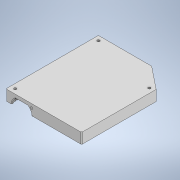
# Autodesk Inventor part: BoxDeckel
Saved by Autodesk Inventor 2020 (Build 240168000, 168)
## iProperties
Created: 2020-04-10
Part Number: BoxDeckel
Material: Generisch
Document SubType Name: Modeling
Designer: Windooof
Density: 1 g/cm^3
Appearance: Vorgabe
Author: Windooof
Autodesk Inventor part; units mm, degrees
ref_plane "YZ Plane" through (0, 0, 0) normal (1, 0, 0) x (0, 1, 0)
ref_plane "XZ Plane" through (0, 0, 0) normal (0, 1, 0) x (-1, 0, 0)
ref_plane "XY Plane" through (0, 0, 0) normal (0, 0, 1) x (1, 0, 0)
sketch "SketchBase" plane through (0, 0, 0) normal (0, 1, 0) x (-1, 0, 0)
  line L0 (45, 55) -> (-45, 55)
  line L1 (-45, 55) -> (-45, -33.701562)
  line L2 (-18.376953, -55) -> (45, -55)
  line L3 (45, -55) -> (45, 55)
  line L4 (63, 0) -> (-63, 0) construction
  line L5 (0, -77) -> (0, 77) construction
  line L6 (42.5, 52.5) -> (-42.5, 52.5)
  line L7 (-42.5, 52.5) -> (-42.5, -32.5)
  line L8 (-17.5, -52.5) -> (42.5, -52.5)
  line L9 (42.5, -52.5) -> (42.5, 52.5)
  line L10 (0.5, 12.5) -> (7.5, 12.5)
  line L11 (0.5, 5.5) -> (0.5, 12.5)
  line L12 (7.5, 5.5) -> (0.5, 5.5)
  line L13 (0.5, 5.5) -> (7.5, 5.5)
  line L14 (0.5, 3.5) -> (0.5, 5.5)
  line L15 (9.5, 12.5) -> (9.5, 3.5)
  line L16 (9.5, 3.5) -> (0.5, 3.5)
  line L17 (7.5, 12.5) -> (9.5, 12.5)
  line L18 (7.5, 12.5) -> (7.5, 5.5)
  line L19 (7.5, 5.5) -> (7.5, 12.5)
  line L20 (2.5, 44.5) -> (7.5, 44.5)
  line L21 (7.5, 44.5) -> (9.5, 44.5)
  line L22 (7.5, 49.5) -> (7.5, 5.5)
  line L23 (2.5, 49.5) -> (2.5, 44.5)
  line L24 (9.5, 44.5) -> (9.5, 49.5)
  line L25 (7.5, 44.5) -> (7.5, 49.5)
  line L26 (7.5, 49.5) -> (7.5, 44.5)
  line L27 (7.5, 49.5) -> (2.5, 49.5)
  line L28 (-42.5, 49.5) -> (7.5, 49.5)
  line L29 (7.5, 5.5) -> (-42.5, 5.5)
  line L30 (-42.5, 5.5) -> (-42.5, 49.5)
  line L31 (-42.5, 49.5) -> (-36.5, 49.5)
  line L32 (-36.5, 49.5) -> (-36.5, 43.5)
  line L33 (-36.5, 43.5) -> (-42.5, 43.5)
  line L34 (-42.5, 43.5) -> (-42.5, 49.5)
  line L35 (-37.5, 5.5) -> (-37.5, 10.5)
  line L36 (-37.5, 5.5) -> (-37.5, 3.5)
  line L37 (-37.5, 10.5) -> (-42.5, 10.5)
  line L38 (-42.5, 10.5) -> (-42.5, 5.5)
  line L39 (-42.5, 5.5) -> (-37.5, 5.5)
  line L40 (-42.5, 5.5) -> (-37.5, 5.5)
  line L41 (-37.5, 3.5) -> (-42.5, 3.5)
  line L42 (-42.5, 3.5) -> (-42.5, 5.5)
  line L43 (-36.5, 49.5) -> (-42.5, 49.5)
  line L44 (-42.5, 49.5) -> (-42.5, 52.5)
  line L45 (-42.5, 52.5) -> (-36.5, 52.5)
  line L46 (-36.5, 52.5) -> (-36.5, 49.5)
  line L47 (2.5, 49.5) -> (2.5, 52.5)
  line L48 (2.5, 52.5) -> (9.5, 52.5)
  line L49 (9.5, 52.5) -> (9.5, 49.5)
  line L50 (-17.5, -52.5) -> (-42.5, -32.5)
  line L51 (-45, -33.701562) -> (-18.376953, -55)
  line L52 (0, -107.8) -> (0, 107.8)
  line L53 (88.2, 0) -> (-88.2, 0)
  point P0 (0, 0)
  point P1 (0, 0)
  point P2 (-45, -55)
  point P3 (-42.5, -52.5)
  dimension "d0" = 110
  dimension "d1" = 90
  dimension "d2" = 2.5
  dimension "d3" = 2.5
  dimension "d4" = 44
  dimension "d5" = 50
  dimension "d6" = 6
  dimension "d7" = 6
  dimension "d8" = 7
  dimension "d9" = 7
  dimension "d10" = 5
  dimension "d11" = 5
  dimension "d12" = 5
  dimension "d13" = 5
  dimension "d14" = 2
  dimension "d15" = 2
  dimension "d16" = 0
  dimension "d17" = 3
  dimension "d18" = 25
  dimension "d19" = 20
  dimension "d20" = 2.5
  constraints: 104 end point, 20 parallel, 13 perpendicular, 11 horizontal, 8 collinear, 5 point on line, 4 other
  measures "d0" distance of L3.start L0.start
  measures "d1" distance of L0.start L0.end
  measures "d2" distance between parallel lines of L0 L6
  measures "d3" distance between parallel lines of L3 L9
  measures "d4" distance of L27.start L12.start
  measures "d5" distance of L12.start L30.start
  measures "d6" distance of L32.start L32.end
  measures "d7" distance of L32.end L33.end
  measures "d8" distance of L10.start L10.end
  measures "d9" distance of L11.start L10.start
  measures "d10" distance of L23.end L21.start
  measures "d11" distance of L27.end L23.end
  measures "d12" distance of L35.start L35.end
  measures "d13" distance of L35.end L38.start
  measures "d14" distance between parallel lines of L16 L13
  measures "d15" distance between parallel lines of L22 L15
  measures "d16" distance between parallel lines of L7 L30
  measures "d17" distance between parallel lines of L6 L28
  measures "d18" distance of L8.start point (-42.5, -52.5)
  measures "d19" distance of L7.end point (-42.5, -52.5)
  measures "d20" distance between parallel lines of L50 L51
extrude "Base" add sketch "SketchBase" along normal blind 2.5
extrude "Walls" add sketch "SketchBase" against normal blind 10 contours L3 L53 L9 L6 L52 L0 | L52 L6 L7 L53 L1 L0 | L3 L2 L52 L8 L9 L53 | L53 L7 L50 L8 L52 L2 L51 L1
sketch "SketchMounts" plane through (0, 0, 0) normal (0, -1, 0) x (1, 0, 0)
  line L0 (-36.5, -46.5) -> (-36.5, -52.5)
  circle A0 centre (-39.5, -49.5) radius 1.5
  line L1 (-42.5, -46.5) -> (-36.5, -46.5)
  line L2 (-36.5, -52.5) -> (-42.5, -46.5) construction
  line L3 (-36.5, -52.5) -> (-42.5, -52.5)
  line L4 (-36.5, -46.5) -> (-42.5, -52.5) construction
  line L5 (-42.5, -52.5) -> (-42.5, -46.5)
  line L6 (36.232693, -29.487776) -> (42.5, -25.843142)
  circle A1 centre (39.5, -31.058125) radius 1.5
  line L7 (42.5, -32.5) -> (36.232693, -29.487776) construction
  line L8 (37.301867, -36.658506) -> (36.232693, -29.487776)
  line L9 (42.5, -32.5) -> (37.301867, -36.658506)
  line L10 (42.5, -25.843142) -> (42.5, -32.5)
  line L11 (-36.5, 52.5) -> (-42.5, 52.5)
  line L12 (-36.5, 46.5) -> (-36.5, 52.5)
  circle A2 centre (-39.5, 49.5) radius 1.5
  line L13 (-42.5, 46.5) -> (-36.5, 46.5)
  line L14 (-42.5, 52.5) -> (-42.5, 46.5)
  line L15 (-42.5, 52.5) -> (-36.5, 46.5) construction
  line L16 (-42.5, 46.5) -> (-36.5, 52.5) construction
  line L17 (42.5, 52.5) -> (42.5, -32.5)
  line L18 (42.5, -32.5) -> (17.5, -52.5)
  line L19 (17.5, -52.5) -> (-42.5, -52.5)
  line L20 (-42.5, -52.5) -> (-42.5, 52.5)
  line L21 (-42.5, 52.5) -> (42.5, 52.5)
  point P0 (0, 0)
  dimension "d81" = 6
  dimension "d82" = 6
  dimension "d83" = 7.25
  dimension "d84" = 7.25
  dimension "d85" = 3
  dimension "d86" = 3
  dimension "d87" = 6
  dimension "d88" = 3
  dimension "d89" = 6
  dimension "d90" = 3
  dimension "d91" = 3
  constraints: 34 end point, 5 collinear, 4 parallel, 3 centre point, 3 midpoint, 3 perpendicular, 2 horizontal, 2 point on line, 1 vertical, 2 other
  measures "d81" distance of L0.start L0.end
  measures "d82" distance of L0.end L3.end
  measures "d83" distance of L6.start L6.end
  measures "d84" distance of L9.end L6.start
  measures "d85" diameter of A0
  measures "d86" diameter of A1
  measures "d87" distance of L12.start L11.start
  measures "d88" diameter of A2
  measures "d89" distance of L11.start L11.end
  measures "d90" distance from line of L6 A1.centre
  measures "d91" distance from line of L10 A1.centre
extrude "Holes" cut sketch "SketchMounts" against normal through all contours A0 | A1 | A2
extrude "Mounts" add sketch "SketchMounts" along normal blind 9 contours L0 L3 L5 L1 | L14 L11 L12 L13 | L8 L6 L10 L9
fillet "RoundingMounts" radius 2 3 edges at (-36.5, -4.5, -46.5) (36.2327, -4.5, -29.4878) (-36.5, -4.5, 46.5)
chamfer "ChamferBase" distance 2 angle 45 13 edges at (-37.0858, 0, -47.0858) (-40.5, 0, -46.5) (-36.5, 0, -50.5) (-9.5, 0, -52.5) (-37.0858, 0, 47.0858) (-36.5, 0, 50.5) (-40.5, 0, 46.5) (42.5, 0, 13.3284) (36.6083, 0, -29.6683) (36.8673, 0, -33.7441) (39.9527, 0, -27.3245) (27.4009, 0, -44.5793) (3, 0, 52.5)
sketch "Skizze2" plane through (-45, 2.5, 55) normal (0, 0, 1) x (1, 0, 0)
  line L0 (34, -27) -> (34, -1)
  circle A0 centre (30.5, -4.5) radius 1.25
  line L1 (18.5, -14) -> (34, -14) construction
  line L2 (18.5, -14) -> (18.5, -27) construction
  circle A1 centre (18.5, -14) radius 12
  line L3 (34, -1) -> (3, -1)
  line L4 (3, -1) -> (3, -27)
  circle A2 centre (6.5, -23.5) radius 1.25
  line L5 (3, -27) -> (34, -27)
  line L6 (0, -2.5) -> (92.252731, -2.5) construction
  line L7 (0, -32.026862) -> (0, -2.5) construction
  line L8 (25.831439, -4.5) -> (11.168561, -4.5)
  line L9 (11.168561, -23.5) -> (25.831439, -23.5)
  line L10 (26.25, -25.5) -> (26.25, -14) construction
  line L11 (26.25, -14) -> (26.25, -2.5) construction
  line L12 (87.5, -2.5) -> (2.5, -2.5)
  line L13 (0, -12.5) -> (0, 0)
  dimension "d25" = 26
  dimension "d26" = 31
  dimension "d27" = 24
  dimension "d28" = 2.5
  dimension "d29" = 2.5
  dimension "d30" = 19
  dimension "d31" = 24
  dimension "d32" = 3.5
  dimension "d33" = 3.5
  dimension "d34" = 3
  dimension "d35" = 1.5
  constraints: 24 end point, 4 point on circle, 3 centre point, 3 collinear, 3 horizontal, 3 midpoint, 3 parallel, 3 point on line, 3 vertical, 1 perpendicular
  measures "d25" distance of L5.end L3.start
  measures "d26" distance of L3.start L4.start
  measures "d27" diameter of A1
  measures "d28" diameter of A0
  measures "d29" diameter of A2
  measures "d30" vertical distance of A2.centre A0.centre
  measures "d31" horizontal distance of A2.centre A0.centre
  measures "d32" distance from line of L3 A0.centre
  measures "d33" distance from line of L0 A0.centre
  measures "d34" distance between parallel lines of L7 L4
  measures "d35" distance between parallel lines of L3 L6
extrude "USB-Cutout" cut sketch "Skizze2" against normal blind 10 contours A1 L9 L8 | A0
sketch "Skizze3" plane through (-45, 2.5, -55) normal (-1, 0, 0) x (0, 0, 1)
  line L0 (15, -17.5) -> (15, -5)
  line L1 (46, -5) -> (46, -17.5)
  circle A0 centre (18.005, -11.25) radius 1.55
  line L2 (21.5, -17.125) -> (20.5, -5.375)
  line L3 (15.173981, -5.375) -> (15.173981, -5) construction
  line L4 (15.821992, -17.125) -> (15.821992, -17.5) construction
  line L5 (30.5, -5) -> (30.5, -17.5) construction
  line L6 (39.5, -17.125) -> (21.5, -17.125)
  line L7 (20.5, -5.375) -> (40.5, -5.375)
  line L8 (46, -17.5) -> (15, -17.5)
  line L9 (46, -11.25) -> (15, -11.25) construction
  line L10 (15, -5) -> (46, -5)
  line L11 (40.5, -5.375) -> (39.5, -17.125)
  circle A1 centre (42.995, -11.25) radius 1.55
  line L12 (0, -21.767357) -> (0, -2.5) construction
  line L13 (0, -2.5) -> (130.232118, -2.5) construction
  line L14 (107.5, -2.5) -> (2.5, -2.5)
  line L15 (0, -12.5) -> (0, 0)
  dimension "d38" = 31
  dimension "d39" = 12.5
  dimension "d40" = 20
  dimension "d41" = 11.75
  dimension "d42" = 18
  dimension "d43" = 3.1
  dimension "d44" = 24.99
  dimension "d45" = 15
  dimension "d46" = 2.5
  constraints: 28 end point, 5 point on line, 4 midpoint, 4 parallel, 3 perpendicular, 2 centre point, 2 collinear, 2 horizontal, 1 equal radius, 2 other
  measures "d38" distance of L0.end L10.end
  measures "d39" distance between parallel lines of L8 L10
  measures "d40" distance of L7.start L7.end
  measures "d41" distance between parallel lines of L6 L7
  measures "d42" distance of L6.start L6.end
  measures "d43" diameter of A0
  measures "d44" distance of A1.centre A0.centre
  measures "d45" distance between parallel lines of L12 L0
  measures "d46" distance between parallel lines of L13 L10
extrude "Stepper-Cutout" cut sketch "Skizze3" against normal blind 2.5 contours A0 | L2 L7 L11 L6 | A1
sketch "Skizze4" plane through (18.376953, 2.5, -55) normal (0, 0, -1) x (-1, 0, 0)
  circle A0 centre (43.126953, -10.25) radius 5.25
  line L0 (63.376953, -2.5) -> (63.376953, -2.5) construction
  line L1 (26.623047, -2.5) -> (63.376953, -2.5) construction
  line L2 (63.376953, -12.5) -> (63.376953, 0)
  line L3 (60.876953, -2.5) -> (0.876953, -2.5)
  dimension "d49" = 10.5
  dimension "d50" = 20.25
  dimension "d51" = 7.75
  constraints: 4 end point, 2 collinear, 1 centre point
  measures "d49" diameter of A0
  measures "d50" distance from line of L0 A0.centre
  measures "d51" distance from line of L1 A0.centre
extrude "Power-Cutout" cut sketch "Skizze4" against normal blind 2.5
chamfer "ChamferOutside" distance 1 angle 45 3 edges at (-45, -3.75, -55) (-45, -3.75, 55) (45, -3.75, 55)
fillet "RoundingCutouts" radius 0.75 8 edges at (-45, -6.4375, -14.8032) (-45, -2.875, -24.5) (-45, -6.4375, -34.1968) (-43.75, -2.875, -34.5) (-43.75, -2.875, -14.5) (-36.9172, -5.5434, 55) (-26.5, -2, 55) (-16.0828, -5.5434, 55)
